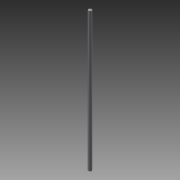
# Autodesk Inventor part: Elevator Drive Shaft
Saved by Autodesk Inventor 2015 (Build 190159000, 159)
## iProperties
Created: 2015-02-06
Part Number: Elevator Drive Shaft
Material: Generic
Document SubType Name: Modeling
Designer: chapale16
Density: 1 g/cm^3
Appearance: Default
Author: chapale16
Autodesk Inventor part; units mm, degrees
ref_plane "YZ Plane" through (0, 0, 0) normal (1, 0, 0) x (0, 1, 0)
ref_plane "XZ Plane" through (0, 0, 0) normal (0, 1, 0) x (-1, 0, 0)
ref_plane "XY Plane" through (0, 0, 0) normal (0, 0, 1) x (1, 0, 0)
sketch "Sketch1" plane through (0, 0, 0) normal (0, 1, 0) x (-1, 0, 0)
  line L0 (-3.6687, -6.3544) -> (-7.3374, 0)
  line L1 (-7.3374, 0) -> (-3.6687, 6.3544)
  line L2 (-3.6687, 6.3544) -> (3.6687, 6.3544)
  line L3 (3.6687, 6.3544) -> (7.3374, 0)
  line L4 (7.3374, 0) -> (3.6687, -6.3544)
  line L5 (3.6687, -6.3544) -> (-3.6687, -6.3544)
  point P0 (0, 0)
  point P1 (0, 0)
  constraints: 12 end point, 1 coincident, 13 other
extrude "Extrusion1" add sketch "Sketch1" along normal blind 591.4136
body "Solid1"
